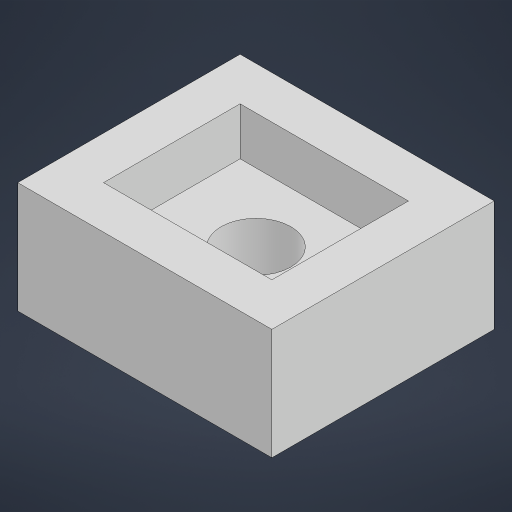
# Autodesk Inventor part: zigu
Saved by Autodesk Inventor 2024.2 (Build 282272000, 272)
## iProperties
Created: 2024-03-13
Part Number: zigu
Material: 一般
Document SubType Name: Modeling
Designer: Hanaoka
Density: 1 g/cm^3
Appearance: 既定
Author: Hanaoka
Autodesk Inventor part; units mm, degrees
ref_plane "YZ Plane" through (0, 0, 0) normal (1, 0, 0) x (0, 1, 0)
ref_plane "XZ Plane" through (0, 0, 0) normal (0, 1, 0) x (-1, 0, 0)
ref_plane "XY Plane" through (0, 0, 0) normal (0, 0, 1) x (1, 0, 0)
sketch "スケッチ1" plane through (0, 0, 0) normal (0, 1, 0) x (-1, 0, 0)
  circle A0 centre (0, 0) radius 1.1
  line L0 (-2.65, 2.15) -> (2.65, 2.15)
  line L1 (2.65, 2.15) -> (2.65, -2.15)
  line L2 (2.65, -2.15) -> (-2.65, -2.15)
  line L3 (-2.65, -2.15) -> (-2.65, 2.15)
  line L4 (-2.65, 2.15) -> (2.65, -2.15) construction
  line L5 (2.65, 2.15) -> (-2.65, -2.15) construction
  line L6 (-4, 3.5) -> (4, 3.5)
  line L7 (4, 3.5) -> (4, -3.5)
  line L8 (4, -3.5) -> (-4, -3.5)
  line L9 (-4, -3.5) -> (-4, 3.5)
  line L10 (-4, 3.5) -> (4, -3.5) construction
  line L11 (4, 3.5) -> (-4, -3.5) construction
  dimension "d0" = 2.2
  dimension "d1" = 5.3
  dimension "d2" = 4.3
  dimension "d3" = 7
  dimension "d4" = 8
  constraints: 24 end point, 4 midpoint, 4 parallel, 2 horizontal, 2 perpendicular, 1 centre point, 1 coincident
  measures "d0" diameter of A0
  measures "d1" distance of L1.end L2.end
  measures "d2" distance of L0.end L1.end
  measures "d3" distance of L6.end L7.end
  measures "d4" distance of L7.end L8.end
extrude "押し出し1" add sketch "スケッチ1" along normal blind 2 contours L0 L1 L2 L3 | L6 L7 L8 L9
extrude "押し出し2" add sketch "スケッチ1" along normal blind 3.5 contours L6 L7 L8 L9
